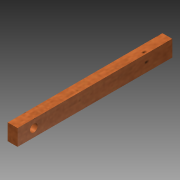
# Autodesk Inventor part: WoodArm
Saved by Autodesk Inventor 2014 SP1 (Build 180222100, 222)
## iProperties
Created: 2015-05-01
Part Number: WoodArm
Material: Wood (Cherry)
Document SubType Name: Modeling
Designer: david
Mass: 3.78 g
Surface Area: 33.2 cm^2
Volume: 6 cm^3
Density: 0.63 g/cm^3
Appearance: Cherry - Natural Low Gloss
Author: david
Autodesk Inventor part; units mm, degrees
ref_plane "YZ Plane" through (0, 0, 0) normal (1, 0, 0) x (0, 1, 0)
ref_plane "XZ Plane" through (0, 0, 0) normal (0, 1, 0) x (-1, 0, 0)
ref_plane "XY Plane" through (0, 0, 0) normal (0, 0, 1) x (1, 0, 0)
sketch "Sketch1" plane through (0, 0, 0) normal (0, 1, 0) x (-1, 0, 0)
  line L0 (-3, -5) -> (3, -5)
  line L1 (3, -5) -> (3, 5)
  line L2 (3, 5) -> (-3, 5)
  line L3 (-3, 5) -> (-3, -5)
  line L4 (-3, -5) -> (3, 5) construction
  line L5 (3, -5) -> (-3, 5) construction
  point P0 (0, 0)
  dimension "d0" = 6
  dimension "d1" = 10
  constraints: 12 end point, 2 midpoint, 2 parallel, 1 horizontal, 1 perpendicular
  measures "d0" distance of L2.end L1.end
  measures "d1" distance of L1.end L0.end
extrude "Extrusion1" add sketch "Sketch1" along normal blind 95
sketch "Sketch2" plane through (-3, 0, -5) normal (-1, 0, 0) x (0, 0, 1)
  line L0 (0, 0) -> (10, 0) projected
  line L1 (0, 0) -> (0, 95) projected
  circle A0 centre (5, 10) radius 2.35
  line L2 (5, 0) -> (5, 20) construction
  dimension "d4" = 4.7
  dimension "d5" = 10
  constraints: 2 end point, 1 centre point, 1 coincident, 1 midpoint, 1 parallel
  measures "d4" diameter of A0
  measures "d5" distance from line of L0 A0.centre
extrude "Extrusion2" cut sketch "Sketch2" against normal up to next
body "Solid1"
